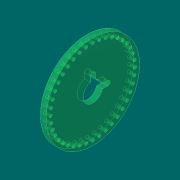
# Autodesk Inventor part: spoolGearSide
Saved by Autodesk Inventor 2016 (Build 200138000, 138)
## iProperties
Created: 2015-10-05
Part Number: spoolGearSide
Material: Polycarbonate, Clear
Document SubType Name: Modeling
Designer: Sawaiz
Density: 1.2 g/cm^3
Appearance: Clear - Green 1
Mass: 43.5641 g
Surface Area: 177.121 cm^2
Volume: 41.0982 cm^3
Author: Sawaiz
Autodesk Inventor part; units mm, degrees
ref_plane "YZ Plane" through (0, 0, 0) normal (1, 0, 0) x (0, 1, 0)
ref_plane "XZ Plane" through (0, 0, 0) normal (0, 1, 0) x (-1, 0, 0)
ref_plane "XY Plane" through (0, 0, 0) normal (0, 0, 1) x (1, 0, 0)
sketch "Sketch2" plane through (0, 0, 0) normal (1, 0, 0) x (0, 1, 0)
  circle A0 centre (0, 0) radius 47.5
  dimension "d7" = 95
  constraints: 1 centre point, 1 coincident
  measures "d7" diameter of A0
extrude "Extrusion1" add sketch "Sketch2" along normal blind 5.588
sketch "Sketch3" plane through (5.588, 0, 0) normal (1, 0, 0) x (0, 0, -1)
  circle A0 centre (0, 0) radius 47.5 projected
  line L0 (0, 0) -> (-47.5, 0)
  circle A1 centre (0, 0) radius 47.5 projected
  point P0 (-42.825, 0)
  dimension "d10" = 42.825
  constraints: 2 end point, 2 horizontal alignment, 1 horizontal, 1 point on line, 2 other
  measures "d10" distance of point (0, 0) point (-42.825, 0)
hole "Hole1" at (5.588, 0, 42.825) direction (-1, 0, 0) diameter 3.1 end through all
pattern_circular "Circular Pattern1" count 40 over 360 about axis through (-10, 0, 0) along (1, 0, 0) of "Hole1"
sketch "Sketch4" plane through (5.588, 0, 0) normal (1, 0, 0) x (0, 0, -1)
  point P0 (0, 0)
  point P1 (0, 0)
  constraints: 1 coincident
hole "Hole2" at (5.588, 0, 0) direction (-1, 0, 0) diameter 20 end through all
sketch "Sketch5" plane through (5.588, 0, 0) normal (1, 0, 0) x (0, 0, -1)
  line L0 (0, -2.5) -> (-15, -2.5)
  line L1 (-15, -2.5) -> (-15, 2.5)
  line L2 (-15, 2.5) -> (0, 2.5)
  line L3 (0, 2.5) -> (0, -2.5)
  line L4 (-2.5, 0) -> (2.5, 0)
  line L5 (2.5, 0) -> (2.5, 15)
  line L6 (2.5, 15) -> (-2.5, 15)
  line L7 (-2.5, 15) -> (-2.5, 0)
  arc A0 (-15, 2.5) -> (-15, -2.5) centre (-15, 0) ccw
  arc A1 (2.5, 15) -> (-2.5, 15) centre (0, 15) ccw
  point P0 (0, 0)
  point P1 (0, 0)
  dimension "d28" = 5
  dimension "d29" = 5
  dimension "d30" = 15
  dimension "d31" = 15
  constraints: 16 end point, 4 parallel, 4 point on circle, 4 tangent, 2 centre point, 2 horizontal, 2 midpoint, 2 perpendicular, 1 coincident
  measures "d28" distance of L4.start L4.end
  measures "d29" distance of L2.end L0.start
  measures "d30" distance between parallel lines of L3 L1
  measures "d31" distance between parallel lines of L4 L6
extrude "Extrusion2" cut sketch "Sketch5" against normal through all
equation "\"d7\" = spoolDiameter"
equation "\"d8\" = spoolThickness"
equation "\"d10\" = -0.5 * cardPinDiameter + 0.5 * spoolDiameter - materialThickness"
equation "\"materialThickness\" = 3.175"
equation "\"laserKerf\" = 0.1"
equation "\"cardPinDiameter\" = 3"
equation "\"spoolDiameter\" = 95"
equation "\"centeralShaftDiameter\" = 8"
equation "\"cardHeight\" = 53.98"
equation "\"cardWidth\" = 85.6"
equation "\"cardThickness\" = 0.76"
equation "\"cardFillet\" = 2.88"
equation "\"cardClearence\" = 0.5"
equation "\"bearingOd\" = 22"
equation "\"bearingWidth\" = 8"
equation "\"axleHeight\" = 95"
equation "\"nutTrapDepth\" = 2.5"
equation "\"nutTrapwidth\" = 5.5"
equation "\"nutTrapClearence\" = 2"
equation "\"magnetDiameter\" = 6"
equation "\"magnetLength\" = 3"
equation "\"magnetProtusion\" = 0.25"
equation "\"spoolThickness\" = 5.588"
body "Solid1"
